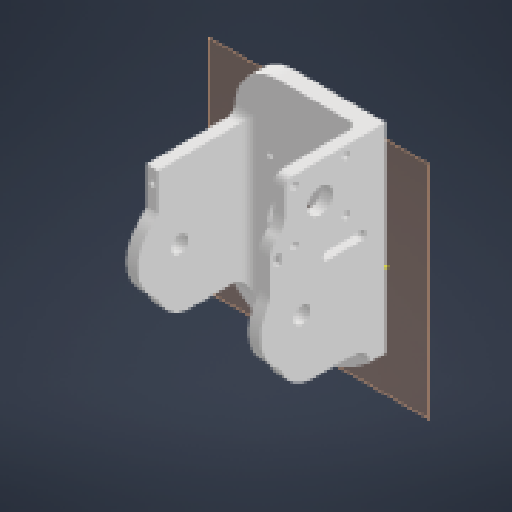
# Autodesk Inventor part: Part1
Saved by Autodesk Inventor 2023 (Build 270158000, 158)
## iProperties
Created: 2023-09-09
Part Number: Part1
Material: Generic
Document SubType Name: Modeling
Designer: philo
Density: 1 g/cm^3
Appearance: Default
Author: philo
Autodesk Inventor part; units mm, degrees
ref_plane "YZ Plane" through (0, 0, 0) normal (1, 0, 0) x (0, 1, 0)
ref_plane "XZ Plane" through (0, 0, 0) normal (0, 1, 0) x (-1, 0, 0)
ref_plane "XY Plane" through (0, 0, 0) normal (0, 0, 1) x (1, 0, 0)
ref_plane "Work Plane1" through (0, 0, 0) normal (0, 0, 1) x (1, 0, 0)
sketch "Sketch1" plane through (0, 0, 0) normal (0, 0, 1) x (1, 0, 0)
  circle A0 centre (-19, 33) radius 1.5
  circle A1 centre (19, -33) radius 1.5
  circle A2 centre (0, 33) radius 1.5
  circle A3 centre (-19, -33) radius 1.5
  circle A4 centre (0, -33) radius 1.5
  circle A5 centre (19, 33) radius 1.5
  circle A6 centre (0, 0) radius 60
  circle A7 centre (8.90567, -8.04295) radius 1.5
  circle A8 centre (8.04295, 8.90567) radius 1.5
  circle A9 centre (-8.04295, -8.90567) radius 1.5
  circle A10 centre (-8.90567, 8.04295) radius 1.5
  circle A11 centre (0, 0) radius 4
  circle A12 centre (-36.92635, 33.711195) radius 1.5
  circle A13 centre (36.92635, -33.711195) radius 1.5
  circle A14 centre (33.711195, 36.92635) radius 1.5
  circle A15 centre (-33.711195, -36.92635) radius 1.5
  line L0 (-40, -63) -> (40, -63)
  line L1 (40, -63) -> (40, 67)
  line L2 (40, 67) -> (-40, 67)
  line L3 (-40, 67) -> (-40, -63)
  point P0 (0, 0)
  point P1 (-40, 44.72136)
  point P2 (-40, -44.72136)
  point P3 (40, -44.72136)
  point P4 (40, 44.72136)
  dimension "d0" = 40
  dimension "d1" = 40
  dimension "d2" = 130
  dimension "d3" = 67
  constraints: 8 end point, 2 parallel, 1 horizontal, 1 perpendicular
  measures "d0" distance from line of L3 point (0, 0)
  measures "d1" distance from line of point (0, 0) L1
  measures "d2" distance between parallel lines of L0 L2
  measures "d3" distance from line of L2 point (0, 0)
extrude "Extrusion1" add sketch "Sketch1" along normal blind 10 contours L1 A6 L3 | A12 | A13 | A14 | A15
sketch "Sketch2" plane through (0, 0, 10) normal (0, 0, 1) x (1, 0, 0)
  circle A0 centre (0, 0) radius 20
  dimension "d6" = 40
  constraints: 1 centre point, 1 coincident
  measures "d6" diameter of A0
extrude "Extrusion2" cut sketch "Sketch2" against normal blind 10
sketch "Sketch3" plane through (0, 0, 10) normal (0, 0, 1) x (1, 0, 0)
  circle A0 centre (0, 0) radius 20
  arc A1 (-40, -44.72136) -> (40, -44.72136) centre (0, 0) ccw
  line L0 (40, -44.72136) -> (40, 44.72136)
  arc A2 (40, 44.72136) -> (-40, 44.72136) centre (0, 0) ccw
  line L1 (-40, 44.72136) -> (-40, -44.72136)
  circle A3 centre (19, 33) radius 1.5
  circle A4 centre (0, -33) radius 1.5
  circle A5 centre (-19, -33) radius 1.5
  circle A6 centre (0, 33) radius 1.5
  circle A7 centre (19, -33) radius 1.5
  circle A8 centre (-19, 33) radius 1.5
  line L2 (-40, -57.711006) -> (-33, -57.711006)
  line L3 (-33, -57.711006) -> (-33, 58.456455)
  line L4 (-33, 58.456455) -> (-40, 58.456455)
  line L5 (-40, 58.456455) -> (-40, -57.711006)
  line L6 (40, -61.156651) -> (33, -61.156651)
  line L7 (33, -61.156651) -> (33, 64.527353)
  line L8 (33, 64.527353) -> (40, 64.527353)
  line L9 (40, 64.527353) -> (40, -61.156651)
  point P0 (33, 50.109879)
  point P1 (33, -50.109879)
  point P2 (-33, -50.109879)
  point P3 (-33, 50.109879)
  dimension "d9" = 7
  dimension "d10" = 7
  constraints: 16 end point, 4 parallel, 2 horizontal, 2 perpendicular, 1 point on line
  measures "d9" distance of L4.end L3.end
  measures "d10" distance of L7.end L8.end
extrude "Extrusion3" add sketch "Sketch3" along normal blind 50 contours L1 A2 L3 A1 | L7 A2 L0 A1
fillet "Fillet1" radius 5 2 edges at (-33, 0, 10) (33, 0, 10)
sketch "Sketch4" plane through (40, -44.72136, 0) normal (1, 0, 0) x (0, 0, -1)
  circle A0 centre (-50, 44.831239) radius 5
  line L0 (-60, 0) -> (-60, 89.442719)
  line L1 (-15, 94.831239) -> (-60, 94.831239)
  point P0 (0, 44.72136)
  dimension "d14" = 10
  dimension "d15" = 10
  dimension "d16" = 50
  constraints: 1 centre point
  measures "d14" diameter of A0
  measures "d15" distance from line of L0 A0.centre
  measures "d16" distance from line of L1 A0.centre
extrude "Extrusion4" cut sketch "Sketch4" against normal blind 200
sketch "Sketch5" plane through (40, -44.72136, 0) normal (1, 0, 0) x (0, 0, -1)
  circle A0 centre (-50, 44.831239) radius 5.5
  circle A1 centre (-50, 44.831239) radius 25
  point P0 (0, 44.72136)
  dimension "d19" = 50
  constraints: 1 centre point, 1 coincident
  measures "d19" diameter of A1
extrude "Extrusion5" add sketch "Sketch5" against normal blind 7
fillet "Fillet2" radius 15 2 edges at (36.5, -22.803, 60) (36.5, 23.0228, 60)
sketch "Sketch6" plane through (40, -44.72136, 0) normal (1, 0, 0) x (0, 0, -1)
  point P0 (0, 44.72136)
sketch "Sketch7" plane through (-40, -44.72136, 0) normal (-1, 0, 0) x (0, 0, 1)
  line L0 (60, 94.831239) -> (60, 76.056229)
  line L1 (15, 94.831239) -> (60, 94.831239)
  line L2 (15, -5.38852) -> (15, 94.831239)
  line L3 (15, -5.38852) -> (60, -5.38852)
  line L4 (60, 13.606249) -> (60, -5.38852)
  arc A0 (65.625, 25.31562) -> (60, 13.606249) centre (75, 13.606249) ccw
  arc A1 (65.625, 25.31562) -> (65.625, 64.346858) centre (50, 44.831239) ccw
  arc A2 (60, 76.056229) -> (65.625, 64.346858) centre (75, 76.056229) ccw
  circle A3 centre (50, 44.831239) radius 5
  circle A4 centre (50, 44.831239) radius 5
  line L5 (0, 89.442719) -> (0, 0)
  line L6 (0, 0) -> (60, 0)
  line L7 (60, 89.442719) -> (60, 0)
  line L8 (0, 89.442719) -> (60, 89.442719)
  point P0 (0, 44.72136)
  point P1 (60, 76.056229)
  point P2 (60, 13.606249)
extrude "Extrusion6" add sketch "Sketch7" against normal blind 7 contours A2 A1 A0 L7
sketch "Sketch9" plane through (0, 0, 0) normal (0, 0, -1) x (-1, 0, 0)
  arc A0 (40, 44.72136) -> (-40, 44.72136) centre (0, 0) ccw
  line L0 (-40, 44.72136) -> (40, 44.72136)
  line L1 (40, 44.72136) -> (40, 74.72136)
  line L2 (40, 74.72136) -> (-40, 74.72136)
  line L3 (-40, 74.72136) -> (-40, 44.72136)
  point P0 (0, 0)
  point P1 (40, 44.72136)
  dimension "d30" = 30
  constraints: 8 end point, 2 parallel, 1 horizontal, 1 perpendicular
  measures "d30" distance of L1.end L0.end
extrude "Extrusion8" add sketch "Sketch9" against normal blind 10 contours A0 L3 L2 L1
sketch "Sketch10" plane through (0, 0, 10) normal (0, 0, 1) x (1, 0, 0)
  line L0 (33, 50.109879) -> (33, 31.334869)
  arc A0 (-28, 53.065997) -> (-40, 44.72136) centre (0, 0) ccw
  line L1 (40, 74.72136) -> (-40, 74.72136)
  line L2 (-40, 44.72136) -> (-33, 44.72136)
  line L3 (-33, 44.72136) -> (-33, 74.72136)
  line L4 (-33, 74.72136) -> (-40, 74.72136)
  line L5 (-40, 74.72136) -> (-40, 44.72136)
  line L6 (40, 44.72136) -> (40, 74.72136)
  line L7 (40, 74.72136) -> (33, 74.72136)
  line L8 (33, 74.72136) -> (33, 44.72136)
  line L9 (33, 44.72136) -> (40, 44.72136)
  line L10 (40, 44.72136) -> (40, 74.72136)
  point P0 (0, 0)
  point P1 (-33, 50.109879)
  dimension "d33" = 7
  constraints: 16 end point, 4 parallel, 2 horizontal, 2 perpendicular, 2 point on line
  measures "d33" distance of L4.end L3.end
extrude "Extrusion9" add sketch "Sketch10" along normal blind 50 contours L8 L1 L6 L9 L0 | A0 L5 L1 L3
sketch "Sketch11" plane through (40, -44.72136, 60) normal (1, 0, 0) x (0, 0, -1)
  line L0 (-1, 80.442719) -> (-1, 116.442719)
  line L1 (-1, 116.442719) -> (3, 120.442719)
  line L2 (3, 120.442719) -> (39, 120.442719)
  line L3 (39, 120.442719) -> (43, 116.442719)
  line L4 (43, 116.442719) -> (43, 80.442719)
  line L5 (43, 80.442719) -> (39, 76.442719)
  line L6 (39, 76.442719) -> (3, 76.442719)
  line L7 (3, 76.442719) -> (-1, 80.442719)
  circle A0 centre (21, 98.442719) radius 4
  circle A1 centre (5.5, 113.942719) radius 2
  circle A2 centre (36.5, 113.942719) radius 2
  circle A3 centre (36.5, 82.942719) radius 2
  circle A4 centre (5.5, 82.942719) radius 2
  circle A5 centre (21, 98.442719) radius 7.5
  point P0 (60, 44.72136)
  dimension "d36" = 15
  constraints: 1 centre point, 1 coincident
  measures "d36" diameter of A5
extrude "Extrusion10" cut sketch "Sketch11" against normal blind 50 contours A0 | A1 | A2 | A3 | A4 | A5
fillet "Fillet3" radius 5 1 edges at (36.5, 74.7214, 60)
sketch "Sketch12" plane through (-40, -44.72136, 0) normal (-1, 0, 0) x (0, 0, 1)
  line L0 (0, 119.442719) -> (60, 119.442719)
  line L1 (10, 97.787356) -> (10, -8.344637)
  line L2 (60, 119.442719) -> (10, 119.442719)
  line L3 (10, 119.442719) -> (10, 89.442719)
  line L4 (10, 89.442719) -> (60, 89.442719)
  line L5 (60, 89.442719) -> (60, 119.442719)
  point P0 (0, 44.72136)
  point P1 (10, 119.442719)
  dimension "d40" = 30
  constraints: 8 end point, 2 parallel, 1 horizontal, 1 perpendicular, 1 point on line
  measures "d40" distance of L3.end L2.end
extrude "Extrusion11" cut sketch "Sketch12" against normal blind 50
fillet "Fillet4" radius 10 1 edges at (-36.5, 44.7214, 60)
fillet "Fillet5" radius 5 1 edges at (33, 62.4156, 10)
fillet "Fillet6" radius 5 1 edges at (-34, 44.7214, 10)
fillet "Fillet7" radius 25.6375 1 edges at (-40, 74.7214, 5)
sketch "Sketch13" plane through (40, -44.72136, 60) normal (1, 0, 0) x (0, 0, -1)
  line L0 (50, -8.344637) -> (50, 94.442719)
  line L1 (50, 8.615977) -> (-2.709272, 8.615977)
  line L2 (-2.709272, 8.615977) -> (-2.709272, -17.877947)
  line L3 (-2.709272, -17.877947) -> (50, -17.877947)
  line L4 (50, -17.877947) -> (50, 8.615977)
  point P0 (60, 44.72136)
  constraints: 8 end point, 2 parallel, 1 horizontal, 1 perpendicular, 1 point on line
extrude "Extrusion12" cut sketch "Sketch13" against normal blind 200
fillet "Fillet8" radius 19.2875 2 edges at (36.5, -36.1054, 60) (-36.5, -36.1054, 60)
fillet "Fillet9" radius 8.175 2 edges at (-34, -36.1054, 10) (34, -36.1054, 10)
sketch "Sketch15" plane through (40, -44.72136, 10) normal (1, 0, 0) x (0, 0, -1)
  line L0 (-53.01, 83.474434) -> (-56.01, 83.474434)
  line L1 (-56.01, 83.474434) -> (-56.01, 77.474434)
  line L2 (-56.01, 77.474434) -> (-53.01, 77.474434)
  line L3 (-53.01, 77.474434) -> (-53.01, 83.474434)
  line L4 (-50, 114.442719) -> (-50, 76.056229)
  arc A0 (-55.625, 64.346858) -> (-55.625, 25.31562) centre (-40, 44.831239) ccw
  line L5 (-50, 90.170323) -> (-59, 90.170323)
  line L6 (-59, 90.170323) -> (-59, 61.079316)
  line L7 (-59, 61.079316) -> (-50, 61.079316)
  line L8 (-50, 61.079316) -> (-50, 90.170323)
  circle A1 centre (-40, 44.831239) radius 5
  circle A2 centre (-44.5, 82.942719) radius 2
  circle A3 centre (-13.5, 113.942719) radius 2
  circle A4 centre (-13.5, 82.942719) radius 2
  circle A5 centre (-44.5, 113.942719) radius 2
  circle A6 centre (-29, 98.442719) radius 7.5
  arc A7 (-51.36627, 19.86096) -> (-33.835566, 8.615977) centre (-33.835566, 27.903477) ccw
  line L9 (-33.835566, 8.615977) -> (-8.175, 8.615977)
  arc A8 (0, 0.440977) -> (-8.175, 8.615977) centre (-8.175, 0.440977) ccw
  line L10 (0, 0.440977) -> (0, 0)
  line L11 (10, 0) -> (0, 0)
  line L12 (10, 0) -> (10, 119.442719)
  line L13 (10, 119.442719) -> (-45, 119.442719)
  arc A9 (-45, 119.442719) -> (-50, 114.442719) centre (-45, 114.442719) ccw
  line L14 (-50, 76.056229) -> (-50, 114.442719)
  arc A10 (-55.625, 64.346858) -> (-50, 76.056229) centre (-65, 76.056229) ccw
  arc A11 (-55.625, 64.346858) -> (-55.625, 25.31562) centre (-40, 44.831239) ccw
  arc A12 (-51.36627, 19.86096) -> (-55.625, 25.31562) centre (-65, 13.606249) ccw
  point P0 (10, 44.72136)
  dimension "d56" = 9
  constraints: 8 end point, 2 parallel, 1 horizontal, 1 perpendicular, 1 point on circle, 1 point on line
  measures "d56" distance of L7.end L6.end
extrude "Extrusion14" add sketch "Sketch15" against normal blind 7 contours L4 A10 A0 L6 L5
fillet "Fillet13" radius 10.9375 3 edges at (36.5, 45.449, 69) (36.5, 16.358, 69) (36.5, 45.449, 60)
sketch "Sketch16" plane through (-40, -44.72136, 0) normal (-1, 0, 0) x (0, 0, 1)
  line L0 (63.01, 88.574434) -> (63.01, 72.474434)
  line L1 (63.01, 72.474434) -> (66.01, 72.474434)
  line L2 (66.01, 72.474434) -> (66.01, 88.574434)
  line L3 (66.01, 88.574434) -> (63.01, 88.574434)
  line L4 (15, 89.442719) -> (50, 89.442719)
  line L5 (43.029112, 89.442719) -> (63.01, 89.442719)
  line L6 (63.01, 89.442719) -> (63.01, 65.03961)
  line L7 (63.01, 65.03961) -> (43.029112, 65.03961)
  line L8 (43.029112, 65.03961) -> (43.029112, 89.442719)
  point P0 (0, 44.72136)
  constraints: 8 end point, 2 parallel, 2 point on line, 1 horizontal, 1 perpendicular
extrude "Extrusion15" add sketch "Sketch16" against normal blind 7 contours L0 L6 L7 L8 L4 L5
sketch "Sketch17" plane through (-40, 22.321551, 63.01) normal (0, 0, 1) x (1, 0, 0)
  circle A0 centre (3.429566, 13.745931) radius 1.5
  point P0 (40, -22.321551)
extrude "Extrusion16" cut sketch "Sketch17" against normal blind 7
sketch "Sketch18" plane through (40, -44.72136, 10) normal (1, 0, 0) x (0, 0, -1)
  line L0 (-27, 65.505232) -> (-2, 65.505232)
  line L1 (-2, 65.505232) -> (-2, 70.505232)
  line L2 (-2, 70.505232) -> (-27, 70.505232)
  line L3 (-27, 70.505232) -> (-27, 65.505232)
  line L4 (10, 0) -> (10, 119.442719)
  point P0 (10, 44.72136)
  dimension "d64" = 25
  dimension "d65" = 5
  dimension "d66" = 12
  constraints: 8 end point, 2 parallel, 1 horizontal, 1 perpendicular
  measures "d64" distance of L2.end L1.end
  measures "d65" distance of L1.end L0.end
  measures "d66" distance between parallel lines of L4 L1
extrude "Extrusion17" cut sketch "Sketch18" against normal blind 10
fillet "Fillet14" radius 2 4 edges at (36.5, 25.7839, 37) (36.5, 20.7839, 37) (36, 20.7839, 12) (36, 25.7839, 12)
body "Solid1"
